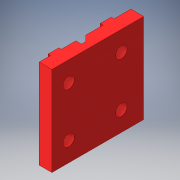
# Autodesk Inventor part: 80-20 extrusion rail
Saved by Autodesk Inventor 2016 SP2 (Build 200236200, 236)
## iProperties
Created: 2018-01-11
Part Number: 80-20 extrusion rail
Material: Generic
Document SubType Name: Modeling
Designer: CAD
Density: 1 g/cm^3
Appearance: Light Red
Author: CAD
Autodesk Inventor part; units mm, degrees
ref_plane "YZ Plane" through (0, 0, 0) normal (1, 0, 0) x (0, 1, 0)
ref_plane "XZ Plane" through (0, 0, 0) normal (0, 1, 0) x (-1, 0, 0)
ref_plane "XY Plane" through (0, 0, 0) normal (0, 0, 1) x (1, 0, 0)
sketch "Sketch1" plane through (0, 0, 0) normal (0, 1, 0) x (-1, 0, 0)
  line L0 (0, 0) -> (0, -51.5938)
  line L1 (0, -51.5938) -> (7.1438, -51.5938)
  line L2 (7.1438, -42.0688) -> (8.7312, -42.0688)
  line L3 (8.7312, -42.0688) -> (8.7312, -35.9728)
  line L4 (8.7312, -35.9728) -> (7.1437, -35.9728)
  line L5 (7.1438, -51.5938) -> (7.1438, -42.0688)
  line L6 (7.1437, -35.9728) -> (7.1437, -26.1938)
  line L7 (0, 0) -> (7.1437, 0)
  line L8 (7.1438, -20.6375) -> (3.9688, -20.6375)
  line L9 (3.9688, -20.6375) -> (3.9688, -23.0188)
  line L10 (3.9688, -23.0188) -> (7.1437, -26.1938)
  line L11 (7.1438, -12.446) -> (8.5408, -12.446)
  line L12 (8.5408, -12.446) -> (8.5408, -6.35)
  line L13 (8.5408, -6.35) -> (7.1438, -6.35)
  line L14 (7.1437, 0) -> (7.1438, -6.35)
  line L15 (7.1438, -12.446) -> (7.1438, -20.6375)
  dimension "d2" = 51.5938
  dimension "d3" = 7.1437
  dimension "d36" = 7.1437
  dimension "d42" = 2.3813
  dimension "d43" = 1.397
  dimension "d44" = 1.397
  dimension "d45" = 6.096
  dimension "d64" = 6.35
  dimension "d65" = 9.525
  dimension "d66" = 6.096
  dimension "d67" = 1.5875
  dimension "d68" = 9.779
  dimension "d69" = 3.9688
  dimension "d71" = 20.6375
  constraints: 32 end point, 11 perpendicular, 3 horizontal, 2 vertical, 1 collinear, 1 parallel
  measures "d2" distance of L0.start L0.end
  measures "d3" distance of L0.end L1.end
  measures "d36" distance of L0.start L7.end
  measures "d42" distance of L8.end L9.end
  measures "d43" distance of L11.start L11.end
  measures "d44" distance of L12.end L13.end
  measures "d45" distance of L11.end L12.end
  measures "d64" distance of L7.end L13.end
  measures "d65" distance between parallel lines of L1 L2
  measures "d66" distance of L2.end L3.end
  measures "d67" distance between parallel lines of L3 L5
  measures "d68" distance from line of L6.end L4
  measures "d69" distance between parallel lines of L0 L9
  measures "d71" distance between parallel lines of L7 L8
extrude "Extrusion1" add sketch "Sketch1" along normal blind 50.292
sketch "Sketch3" plane through (-8.7312, 0, -42.0688) normal (-1, 0, 0) x (0, 0, 1)
  line L0 (6.096, 0) -> (6.096, 50.292) projected
  line L1 (0, 50.292) -> (6.096, 50.292) projected
  line L2 (0, 0) -> (6.096, 0) projected
  line L3 (35.7188, 0) -> (35.7188, 50.292) projected
  point P0 (42.0688, 0)
  point P1 (3.048, 39.1795)
  point P2 (3.048, 11.1125)
  point P3 (32.6708, 39.1795)
  point P4 (32.6708, 11.1125)
  dimension "d49" = 3.048
  dimension "d50" = 3.048
  dimension "d51" = 11.1125
  dimension "d52" = 11.1125
  dimension "d60" = 3.048
  dimension "d61" = 3.048
  dimension "d62" = 0
  dimension "d63" = 0
  measures "d49" distance from line of point (3.048, 39.18) L0
  measures "d50" distance from line of L0 point (3.048, 11.113)
  measures "d51" distance from line of L1 point (3.048, 39.18)
  measures "d52" distance from line of L2 point (3.048, 11.113)
  measures "d60" distance from line of L3 point (32.671, 11.113)
  measures "d61" distance from line of L3 point (32.671, 39.18)
  measures "d62" vertical distance of point (3.048, 39.18) point (32.671, 39.18)
  measures "d63" vertical distance of point (3.048, 11.113) point (32.671, 11.113)
hole "Hole2" at (-8.7312, 39.1795, -39.0208) at (-8.7312, 11.1125, -39.0208) at (-8.7312, 39.1795, -9.398) at (-8.7312, 11.1125, -9.398) direction (1, 0, 0) diameter 6.35 end through all
equation "\"d36\" = d3"
equation "\"d43\" = d14"
equation "\"d44\" = d14"
equation "\"d45\" = d15"
equation "\"d14\" = 1.397"
equation "\"d15\" = 6.096"
body "Solid1"
